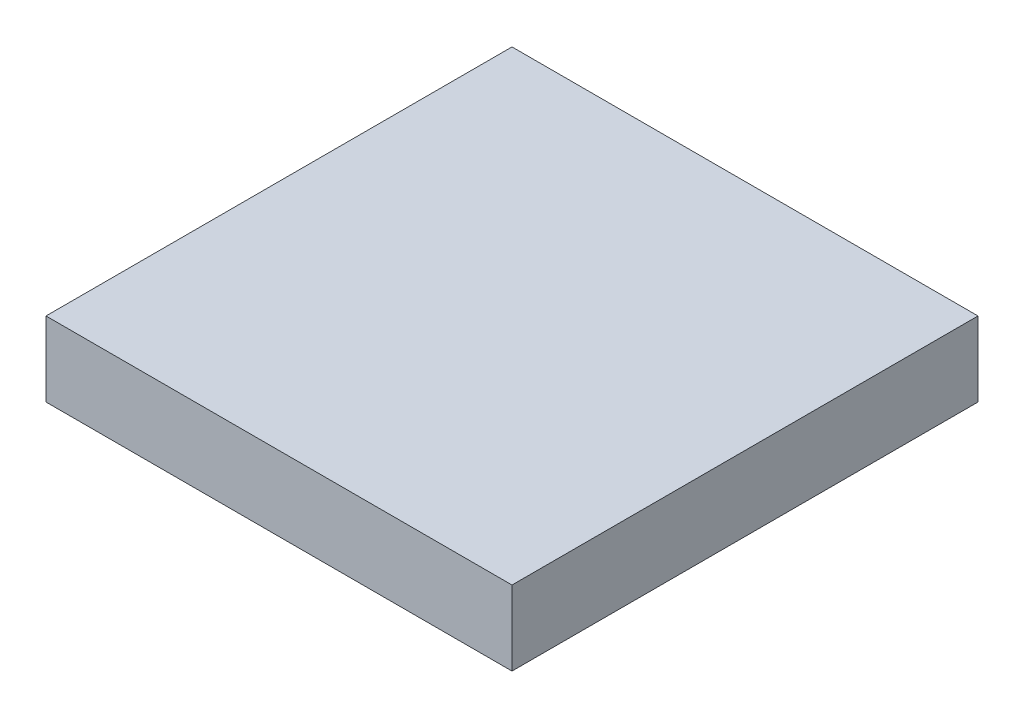
# Autodesk Inventor part: ступица
Saved by Autodesk Inventor 2024.2 (Build 282272000, 272)
## iProperties
Created: 2025-12-13
Part Number: ступица
Material: Типовые
Document SubType Name: Modeling
Designer: katya_notebook
Density: 1 g/cm^3
Appearance: По умолчанию
Author: katya_notebook
Autodesk Inventor part; units mm, degrees
ref_plane "YZ Plane" through (0, 0, 0) normal (1, 0, 0) x (0, 1, 0)
ref_plane "XZ Plane" through (0, 0, 0) normal (0, 1, 0) x (-1, 0, 0)
ref_plane "XY Plane" through (0, 0, 0) normal (0, 0, 1) x (1, 0, 0)
ref_plane "РабПлоскость1" through (-494.6563, -250.4031, -64.2735) normal (0, 1, 0) x (-1, 0, 0)
sketch "Эскиз1" plane through (-494.6563, -250.4031, -64.2735) normal (0, 1, 0) x (-1, 0, 0)
  line L0 (-58.2792, -101.5) -> (58.5237, -101.5) projected
  line L1 (22.5, 91.5) -> (22.5, -91.5) projected
  line L2 (22.5, -101.5) -> (47.5, -101.5)
  line L3 (47.5, -101.5) -> (47.5, -76.5)
  line L4 (47.5, -76.5) -> (22.5, -76.5)
  line L5 (22.5, -76.5) -> (22.5, -101.5)
  point P0 (-494.6563, 64.2735)
  point P1 (22.5, -91.5)
  point P2 (47.5, -101.5)
  point P3 (22.5, -76.5)
  dimension "d0" = 25
  dimension "d1" = 25
  constraints: 8 end point, 2 parallel, 1 horizontal, 1 perpendicular, 1 point on line, 1 other
  measures "d0" distance of L4.end L2.start
  measures "d1" distance of L3.end L4.end
extrude "Выдавливание1" add sketch "Эскиз1" along normal blind 4
